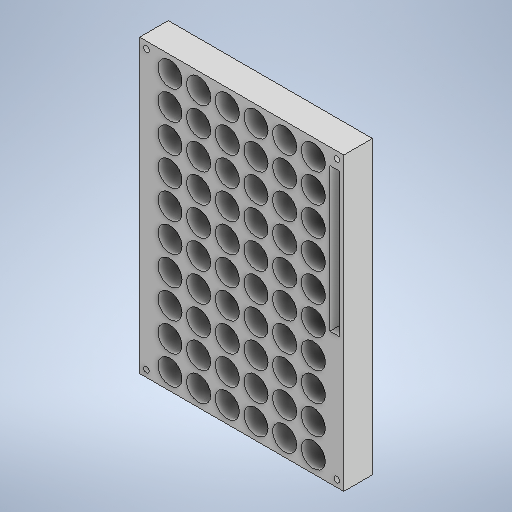
# Autodesk Inventor part: Battery Holder pt1
Saved by Autodesk Inventor 2025.2 (Build 292293000, 293)
## iProperties
Created: 2025-03-23
Part Number: Battery Holder pt1
Material: Generic
Document SubType Name: Modeling
Designer: Mathias
Density: 1 g/cm^3
Appearance: Default
Author: Mathias
Autodesk Inventor part; units mm, degrees
ref_plane "YZ Plane" through (0, 0, 0) normal (1, 0, 0) x (0, 1, 0)
ref_plane "XZ Plane" through (0, 0, 0) normal (0, 1, 0) x (-1, 0, 0)
ref_plane "XY Plane" through (0, 0, 0) normal (0, 0, 1) x (1, 0, 0)
sketch "Sketch1" plane through (0, 0, 0) normal (0, 0, 1) x (1, 0, 0)
  line L0 (0, 0) -> (178, 0)
  line L1 (178, 0) -> (178, 254)
  line L2 (178, 254) -> (0, 254)
  line L3 (0, 254) -> (0, 0)
  circle A0 centre (26.5, 14.5) radius 10.5
  circle A1 centre (26.5, 39.5) radius 10.5
  circle A2 centre (26.5, 64.5) radius 10.5
  circle A3 centre (26.5, 89.5) radius 10.5
  circle A4 centre (26.5, 114.5) radius 10.5
  circle A5 centre (26.5, 139.5) radius 10.5
  circle A6 centre (26.5, 164.5) radius 10.5
  circle A7 centre (26.5, 189.5) radius 10.5
  circle A8 centre (26.5, 214.5) radius 10.5
  circle A9 centre (26.5, 239.5) radius 10.5
  circle A10 centre (51.5, 14.5) radius 10.5
  circle A11 centre (51.5, 39.5) radius 10.5
  circle A12 centre (51.5, 64.5) radius 10.5
  circle A13 centre (51.5, 89.5) radius 10.5
  circle A14 centre (51.5, 114.5) radius 10.5
  circle A15 centre (51.5, 139.5) radius 10.5
  circle A16 centre (51.5, 164.5) radius 10.5
  circle A17 centre (51.5, 189.5) radius 10.5
  circle A18 centre (51.5, 214.5) radius 10.5
  circle A19 centre (51.5, 239.5) radius 10.5
  circle A20 centre (76.5, 14.5) radius 10.5
  circle A21 centre (76.5, 39.5) radius 10.5
  circle A22 centre (76.5, 64.5) radius 10.5
  circle A23 centre (76.5, 89.5) radius 10.5
  circle A24 centre (76.5, 114.5) radius 10.5
  circle A25 centre (76.5, 139.5) radius 10.5
  circle A26 centre (76.5, 164.5) radius 10.5
  circle A27 centre (76.5, 189.5) radius 10.5
  circle A28 centre (76.5, 214.5) radius 10.5
  circle A29 centre (76.5, 239.5) radius 10.5
  circle A30 centre (101.5, 14.5) radius 10.5
  circle A31 centre (101.5, 39.5) radius 10.5
  circle A32 centre (101.5, 64.5) radius 10.5
  circle A33 centre (101.5, 89.5) radius 10.5
  circle A34 centre (101.5, 114.5) radius 10.5
  circle A35 centre (101.5, 139.5) radius 10.5
  circle A36 centre (101.5, 164.5) radius 10.5
  circle A37 centre (101.5, 189.5) radius 10.5
  circle A38 centre (101.5, 214.5) radius 10.5
  circle A39 centre (101.5, 239.5) radius 10.5
  circle A40 centre (126.5, 14.5) radius 10.5
  circle A41 centre (126.5, 39.5) radius 10.5
  circle A42 centre (126.5, 64.5) radius 10.5
  circle A43 centre (126.5, 89.5) radius 10.5
  circle A44 centre (126.5, 114.5) radius 10.5
  circle A45 centre (126.5, 139.5) radius 10.5
  circle A46 centre (126.5, 164.5) radius 10.5
  circle A47 centre (126.5, 189.5) radius 10.5
  circle A48 centre (126.5, 214.5) radius 10.5
  circle A49 centre (126.5, 239.5) radius 10.5
  circle A50 centre (151.5, 14.5) radius 10.5
  circle A51 centre (151.5, 39.5) radius 10.5
  circle A52 centre (151.5, 64.5) radius 10.5
  circle A53 centre (151.5, 89.5) radius 10.5
  circle A54 centre (151.5, 114.5) radius 10.5
  circle A55 centre (151.5, 139.5) radius 10.5
  circle A56 centre (151.5, 164.5) radius 10.5
  circle A57 centre (151.5, 189.5) radius 10.5
  circle A58 centre (151.5, 214.5) radius 10.5
  circle A59 centre (151.5, 239.5) radius 10.5
  circle A60 centre (6, 6) radius 2.5
  circle A61 centre (6, 248) radius 2.5
  circle A62 centre (172, 6) radius 2.5
  circle A63 centre (172, 248) radius 2.5
  line L4 (166, 240) -> (174.5, 240)
  line L5 (174.5, 240) -> (174.5, 115)
  line L6 (174.5, 115) -> (166, 115)
  line L7 (166, 115) -> (166, 240)
  dimension "d0" = 178
  dimension "d1" = 254
  dimension "d2" = 21
  dimension "d5" = 25
  dimension "d8" = 25
  dimension "d11" = 5
  dimension "d12" = 5
  dimension "d13" = 5
  dimension "d14" = 5
  dimension "d15" = 125
  constraints: 64 centre point, 16 end point, 4 perpendicular, 3 horizontal, 2 parallel, 1 vertical, 118 other
  measures "d0" distance of L0.start L0.end
  measures "d1" distance of L0.end L1.end
  measures "d2" diameter of A0
  measures "d5" distance of A0.centre A1.centre
  measures "d8" distance of A0.centre A10.centre
  measures "d11" diameter of A60
  measures "d12" diameter of A61
  measures "d13" diameter of A62
  measures "d14" diameter of A63
  measures "d15" distance of L4.end L5.end
extrude "Extrusion1" add sketch "Sketch1" along normal blind 20
sketch "Sketch2" plane through (0, 0, 0) normal (0, 0, -1) x (-1, 0, 0)
  line L0 (-178, 0) -> (-178, 254) projected
  line L1 (-178, 254) -> (0, 254)
  line L2 (0, 254) -> (0, 0)
  line L3 (0, 0) -> (-178, 0)
  line L4 (-178, 0) -> (-178, 254)
  line L5 (-174.5, 240) -> (-174.5, 115) projected
  line L6 (-166, 115) -> (-166, 240) projected
  line L7 (-174.5, 115) -> (-166, 115)
  line L8 (-166, 115) -> (-166, 125)
  line L9 (-166, 125) -> (-174.5, 125)
  line L10 (-174.5, 125) -> (-174.5, 115)
  line L11 (-161, 5) -> (-92, 5)
  line L12 (-92, 5) -> (-92, 49)
  line L13 (-92, 49) -> (-161, 49)
  line L14 (-161, 49) -> (-161, 5)
  line L15 (-161, 99) -> (-161, 55)
  line L16 (-92, 99) -> (-161, 99)
  line L17 (-92, 55) -> (-92, 99)
  line L18 (-161, 55) -> (-92, 55)
  line L19 (-161, 149) -> (-161, 105)
  line L20 (-92, 149) -> (-161, 149)
  line L21 (-92, 105) -> (-92, 149)
  line L22 (-161, 105) -> (-92, 105)
  line L23 (-161, 199) -> (-161, 155)
  line L24 (-92, 199) -> (-161, 199)
  line L25 (-92, 155) -> (-92, 199)
  line L26 (-161, 155) -> (-92, 155)
  line L27 (-161, 249) -> (-161, 205)
  line L28 (-92, 249) -> (-161, 249)
  line L29 (-92, 205) -> (-92, 249)
  line L30 (-161, 205) -> (-92, 205)
  line L31 (-86, 49) -> (-86, 5)
  line L32 (-17, 49) -> (-86, 49)
  line L33 (-17, 5) -> (-17, 49)
  line L34 (-86, 5) -> (-17, 5)
  line L35 (-86, 99) -> (-86, 55)
  line L36 (-17, 99) -> (-86, 99)
  line L37 (-17, 55) -> (-17, 99)
  line L38 (-86, 55) -> (-17, 55)
  line L39 (-86, 149) -> (-86, 105)
  line L40 (-17, 149) -> (-86, 149)
  line L41 (-17, 105) -> (-17, 149)
  line L42 (-86, 105) -> (-17, 105)
  line L43 (-86, 199) -> (-86, 155)
  line L44 (-17, 199) -> (-86, 199)
  line L45 (-17, 155) -> (-17, 199)
  line L46 (-86, 155) -> (-17, 155)
  line L47 (-86, 249) -> (-86, 205)
  line L48 (-17, 249) -> (-86, 249)
  line L49 (-17, 205) -> (-17, 249)
  line L50 (-86, 205) -> (-17, 205)
  circle A0 centre (-172, 6) radius 2.5 projected
  circle A1 centre (-172, 6) radius 2.5
  circle A2 centre (-172, 248) radius 2.5 projected
  circle A3 centre (-172, 248) radius 2.5
  circle A4 centre (-6, 248) radius 2.5 projected
  circle A5 centre (-6, 248) radius 2.5
  circle A6 centre (-6, 6) radius 2.5 projected
  circle A7 centre (-6, 6) radius 2.5
  dimension "d18" = 10
  dimension "d19" = 69
  dimension "d20" = 44
  dimension "d23" = 50
  dimension "d26" = 75
  constraints: 96 end point, 6 parallel, 4 centre point, 4 coincident, 4 horizontal, 3 perpendicular, 1 point on line, 1 vertical, 72 other
  measures "d18" distance of L8.end L7.end
  measures "d19" distance of L13.end L12.end
  measures "d20" distance of L12.end L11.end
  measures "d23" distance of L13.end L15.start
  measures "d26" distance of L13.end L31.start
extrude "Extrusion2" add sketch "Sketch2" along normal blind 5
body "Solid1"
